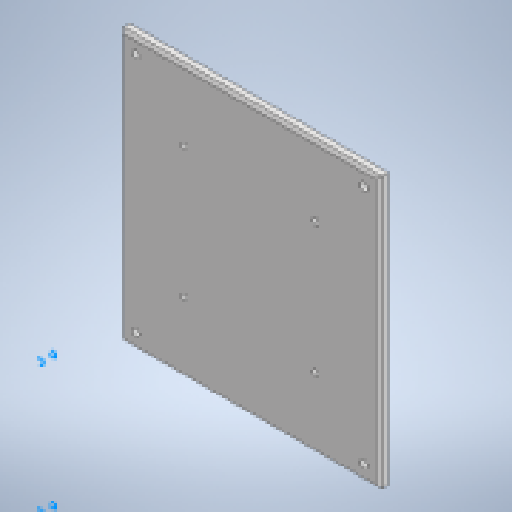
# Autodesk Inventor part: support lidar
Saved by Autodesk Inventor 2024 (Build 280153000, 153)
## iProperties
Created: 2024-03-28
Part Number: support lidar
Material: Générique
Document SubType Name: Modeling
Designer: phaly
Density: 1 g/cm^3
Appearance: Par défaut
Author: phaly
Autodesk Inventor part; units mm, degrees
ref_plane "YZ Plane" through (0, 0, 0) normal (1, 0, 0) x (0, 1, 0)
ref_plane "XZ Plane" through (0, 0, 0) normal (0, 1, 0) x (-1, 0, 0)
ref_plane "XY Plane" through (0, 0, 0) normal (0, 0, 1) x (1, 0, 0)
sketch "Esquisse1" plane through (0, 0, 0) normal (0, 0, 1) x (1, 0, 0)
  line L0 (0, 89) -> (85, 89)
  line L1 (85, 89) -> (85, 0)
  line L2 (85, 0) -> (0, 0)
  line L3 (0, 0) -> (0, 89)
  line L4 (-17.3397, 0) -> (102.0566, 0) projected
  line L5 (0, -18.665) -> (0, 106.9442) projected
  point P0 (0, 0)
  dimension "d0" = 85
  dimension "d1" = 89
  constraints: 8 end point, 2 collinear, 2 parallel, 1 horizontal, 1 perpendicular
  measures "d0" distance of L0.start L0.end
  measures "d1" distance between parallel lines of L2 L0
extrude "Extrusion1" add sketch "Esquisse1" along normal blind 4
sketch "Esquisse2" plane through (0, 0, 4) normal (0, 0, 1) x (1, 0, 0)
  line L0 (85, 0) -> (85, 89) projected
  line L1 (0, 89) -> (0, 0) projected
  line L2 (85, 89) -> (0, 89) projected
  line L3 (0, 0) -> (85, 0) projected
  point P0 (5, 84)
  point P1 (80, 84)
  point P2 (80, 5)
  point P3 (5, 5)
  dimension "d16" = 75
  dimension "d17" = 75
  dimension "d18" = 79
  dimension "d19" = 79
  dimension "d20" = 5
  dimension "d21" = 5
  dimension "d22" = 5
  dimension "d23" = 5
  measures "d16" distance of point (80, 84) point (5, 84)
  measures "d17" distance of point (5, 5) point (80, 5)
  measures "d18" distance of point (80, 84) point (80, 5)
  measures "d19" distance of point (5, 5) point (5, 84)
  measures "d20" distance from line of L0 point (80, 84)
  measures "d21" distance from line of L1 point (5, 5)
  measures "d22" distance from line of L3 point (5, 5)
  measures "d23" distance from line of L2 point (80, 84)
hole "Perçage1" at (5, 84, 4) at (80, 84, 4) at (80, 5, 4) at (5, 5, 4) direction (0, 0, -1) diameter 2.5 end through all
sketch "Esquisse3" plane through (0, 0, 0) normal (0, 0, -1) x (-1, 0, 0)
  line L0 (0, 0) -> (0, 89) projected
  line L1 (0, 89) -> (-85, 89) projected
  point P0 (-21, 66)
  point P1 (-21, 23)
  point P2 (-64, 23)
  point P3 (-64, 66)
  dimension "d32" = 43
  dimension "d33" = 43
  dimension "d34" = 43
  dimension "d35" = 43
  dimension "d36" = 21
  dimension "d44" = 21
  dimension "d45" = 23
  dimension "d46" = 23
  measures "d32" distance of point (-21, 23) point (-21, 66)
  measures "d33" distance of point (-64, 23) point (-64, 66)
  measures "d34" distance of point (-21, 66) point (-64, 66)
  measures "d35" distance of point (-21, 23) point (-64, 23)
  measures "d36" distance from line of L0 point (-21, 66)
  measures "d44" distance from line of L0 point (-21, 23)
  measures "d45" distance from line of L1 point (-64, 66)
  measures "d46" distance from line of L1 point (-21, 66)
hole "Perçage2" at (21, 66, 0) at (21, 23, 0) at (64, 23, 0) at (64, 66, 0) direction (0, 0, 1) diameter 2 end through all
chamfer "Chanfrein1" distance 1 angle 45 8 edges at (42.5, 0, 0) (42.5, 0, 4) (85, 44.5, 0) (42.5, 89, 0) (0, 44.5, 0) (0, 44.5, 4) (85, 44.5, 4) (42.5, 89, 4)
equation "\"d17\" = d16"
equation "\"d19\" = d18"
equation "\"d21\" = d20"
equation "\"d22\" = d21"
equation "\"d23\" = d20"
equation "\"d33\" = d32"
equation "\"d34\" = d33"
equation "\"d35\" = d33"
equation "\"d44\" = d36"
equation "\"d46\" = d45"
